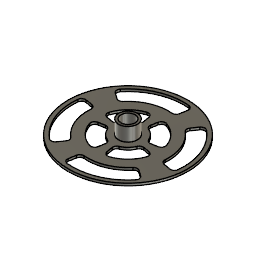
Holder 2 (Autodesk Fusion 360 design; units mm, degrees)
Autodesk Fusion 360 part; units mm, degrees
note: some values were not read from the file. Set by a fixed rule: which sketch regions a step uses.
sketch "Sketch1" plane through (0, 0, 0) normal (0, 0, 1) x (1, 0, 0)
  circle A0 centre (0, 0) radius 75
  circle A1 centre (0, 0) radius 46
  circle A2 centre (0, 0) radius 43
  circle A3 centre (0, 0) radius 11.9
  circle A4 centre (0, 0) radius 8.9
  line L0 (0, 90) -> (0, -90)
  line L1 (12.1554, 68.9365) -> (13.0236, 73.8606)
  line L2 (8.8561, 50.2252) -> (12.1554, 68.9365)
  line L3 (-12.1554, 68.9365) -> (-13.0236, 73.8606)
  line L4 (-8.8561, 50.2252) -> (-12.1554, 68.9365)
  arc A5 (-8.8561, 50.2252) -> (8.8561, 50.2252) centre (0, 0) ccw
  arc A6 (0, 51) -> (-8.8561, 50.2252) centre (0, 0) ccw
  arc A7 (8.8561, 50.2252) -> (0, 51) centre (0, 0) ccw
  arc A8 (-12.1554, 68.9365) -> (12.1554, 68.9365) centre (0, 0) ccw
  arc A9 (12.1554, 68.9365) -> (0, 70) centre (0, 0) ccw
  arc A10 (0, 70) -> (-12.1554, 68.9365) centre (0, 0) ccw
  arc A11 (-6.5986, 37.4227) -> (6.5986, 37.4227) centre (0, 0) ccw
  arc A12 (6.5986, 37.4227) -> (0, 38) centre (0, 0) ccw
  arc A13 (0, 38) -> (-6.5986, 37.4227) centre (0, 0) ccw
  line L5 (0, 0) -> (3.473, 19.6962)
  line L6 (6.5986, 37.4227) -> (8.8561, 50.2252)
  line L7 (3.473, 19.6962) -> (6.5986, 37.4227)
  line L8 (0, 0) -> (-3.473, 19.6962)
  line L9 (-6.5986, 37.4227) -> (-8.8561, 50.2252)
  line L10 (-3.473, 19.6962) -> (-6.5986, 37.4227)
  arc A14 (-3.473, 19.6962) -> (3.473, 19.6962) centre (0, 0) ccw
  arc A15 (0, 20) -> (-3.473, 19.6962) centre (0, 0) ccw
  arc A16 (3.473, 19.6962) -> (0, 20) centre (0, 0) ccw
  arc A17 (-40.1504, 57.3406) -> (-49.4975, 49.4975) centre (0, 0) ccw
  arc A18 (-49.4975, 49.4975) -> (-57.3406, 40.1504) centre (0, 0) ccw
  line L11 (-29.2524, 41.7768) -> (-40.1504, 57.3406)
  arc A19 (-29.2524, 41.7768) -> (-36.0624, 36.0624) centre (0, 0) ccw
  arc A20 (-36.0624, 36.0624) -> (-41.7768, 29.2524) centre (0, 0) ccw
  line L12 (-41.7768, 29.2524) -> (-57.3406, 40.1504)
  arc A21 (-21.7959, 31.1278) -> (-26.8701, 26.8701) centre (0, 0) ccw
  line L13 (-11.4715, 16.383) -> (-21.7959, 31.1278)
  arc A22 (-11.4715, 16.383) -> (-14.1421, 14.1421) centre (0, 0) ccw
  arc A23 (-14.1421, 14.1421) -> (-16.383, 11.4715) centre (0, 0) ccw
  line L14 (-16.383, 11.4715) -> (-31.1278, 21.7959)
  arc A24 (-26.8701, 26.8701) -> (-31.1278, 21.7959) centre (0, 0) ccw
  arc A25 (-68.9365, 12.1554) -> (-70, 0) centre (0, 0) ccw
  arc A26 (-70, 0) -> (-68.9365, -12.1554) centre (0, 0) ccw
  line L15 (-50.2252, 8.8561) -> (-68.9365, 12.1554)
  arc A27 (-50.2252, 8.8561) -> (-51, 0) centre (0, 0) ccw
  arc A28 (-51, 0) -> (-50.2252, -8.8561) centre (0, 0) ccw
  line L16 (-50.2252, -8.8561) -> (-68.9365, -12.1554)
  arc A29 (-37.4227, 6.5986) -> (-38, 0) centre (0, 0) ccw
  line L17 (-19.6962, 3.473) -> (-37.4227, 6.5986)
  arc A30 (-19.6962, 3.473) -> (-20, 0) centre (0, 0) ccw
  arc A31 (-20, 0) -> (-19.6962, -3.473) centre (0, 0) ccw
  line L18 (-19.6962, -3.473) -> (-37.4227, -6.5986)
  arc A32 (-38, 0) -> (-37.4227, -6.5986) centre (0, 0) ccw
  arc A33 (-57.3406, -40.1504) -> (-49.4975, -49.4975) centre (0, 0) ccw
  arc A34 (-49.4975, -49.4975) -> (-40.1504, -57.3406) centre (0, 0) ccw
  line L19 (-41.7768, -29.2524) -> (-57.3406, -40.1504)
  arc A35 (-41.7768, -29.2524) -> (-36.0624, -36.0624) centre (0, 0) ccw
  arc A36 (-36.0624, -36.0624) -> (-29.2524, -41.7768) centre (0, 0) ccw
  line L20 (-29.2524, -41.7768) -> (-40.1504, -57.3406)
  arc A37 (-31.1278, -21.7959) -> (-26.8701, -26.8701) centre (0, 0) ccw
  line L21 (-16.383, -11.4715) -> (-31.1278, -21.7959)
  arc A38 (-16.383, -11.4715) -> (-14.1421, -14.1421) centre (0, 0) ccw
  arc A39 (-14.1421, -14.1421) -> (-11.4715, -16.383) centre (0, 0) ccw
  line L22 (-11.4715, -16.383) -> (-21.7959, -31.1278)
  arc A40 (-26.8701, -26.8701) -> (-21.7959, -31.1278) centre (0, 0) ccw
  arc A41 (-12.1554, -68.9365) -> (0, -70) centre (0, 0) ccw
  arc A42 (0, -70) -> (12.1554, -68.9365) centre (0, 0) ccw
  line L23 (-8.8561, -50.2252) -> (-12.1554, -68.9365)
  arc A43 (-8.8561, -50.2252) -> (0, -51) centre (0, 0) ccw
  arc A44 (0, -51) -> (8.8561, -50.2252) centre (0, 0) ccw
  line L24 (8.8561, -50.2252) -> (12.1554, -68.9365)
  arc A45 (-6.5986, -37.4227) -> (0, -38) centre (0, 0) ccw
  line L25 (-3.473, -19.6962) -> (-6.5986, -37.4227)
  arc A46 (-3.473, -19.6962) -> (0, -20) centre (0, 0) ccw
  arc A47 (0, -20) -> (3.473, -19.6962) centre (0, 0) ccw
  line L26 (3.473, -19.6962) -> (6.5986, -37.4227)
  arc A48 (0, -38) -> (6.5986, -37.4227) centre (0, 0) ccw
  arc A49 (40.1504, -57.3406) -> (49.4975, -49.4975) centre (0, 0) ccw
  arc A50 (49.4975, -49.4975) -> (57.3406, -40.1504) centre (0, 0) ccw
  line L27 (29.2524, -41.7768) -> (40.1504, -57.3406)
  arc A51 (29.2524, -41.7768) -> (36.0624, -36.0624) centre (0, 0) ccw
  arc A52 (36.0624, -36.0624) -> (41.7768, -29.2524) centre (0, 0) ccw
  line L28 (41.7768, -29.2524) -> (57.3406, -40.1504)
  arc A53 (21.7959, -31.1278) -> (26.8701, -26.8701) centre (0, 0) ccw
  line L29 (11.4715, -16.383) -> (21.7959, -31.1278)
  arc A54 (11.4715, -16.383) -> (14.1421, -14.1421) centre (0, 0) ccw
  arc A55 (14.1421, -14.1421) -> (16.383, -11.4715) centre (0, 0) ccw
  line L30 (16.383, -11.4715) -> (31.1278, -21.7959)
  arc A56 (26.8701, -26.8701) -> (31.1278, -21.7959) centre (0, 0) ccw
  arc A57 (68.9365, -12.1554) -> (70, 0) centre (0, 0) ccw
  arc A58 (70, 0) -> (68.9365, 12.1554) centre (0, 0) ccw
  line L31 (50.2252, -8.8561) -> (68.9365, -12.1554)
  arc A59 (50.2252, -8.8561) -> (51, 0) centre (0, 0) ccw
  arc A60 (51, 0) -> (50.2252, 8.8561) centre (0, 0) ccw
  line L32 (50.2252, 8.8561) -> (68.9365, 12.1554)
  arc A61 (37.4227, -6.5986) -> (38, 0) centre (0, 0) ccw
  line L33 (19.6962, -3.473) -> (37.4227, -6.5986)
  arc A62 (19.6962, -3.473) -> (20, 0) centre (0, 0) ccw
  arc A63 (20, 0) -> (19.6962, 3.473) centre (0, 0) ccw
  line L34 (19.6962, 3.473) -> (37.4227, 6.5986)
  arc A64 (38, 0) -> (37.4227, 6.5986) centre (0, 0) ccw
  arc A65 (57.3406, 40.1504) -> (49.4975, 49.4975) centre (0, 0) ccw
  arc A66 (49.4975, 49.4975) -> (40.1504, 57.3406) centre (0, 0) ccw
  line L35 (41.7768, 29.2524) -> (57.3406, 40.1504)
  arc A67 (41.7768, 29.2524) -> (36.0624, 36.0624) centre (0, 0) ccw
  arc A68 (36.0624, 36.0624) -> (29.2524, 41.7768) centre (0, 0) ccw
  line L36 (29.2524, 41.7768) -> (40.1504, 57.3406)
  arc A69 (31.1278, 21.7959) -> (26.8701, 26.8701) centre (0, 0) ccw
  line L37 (16.383, 11.4715) -> (31.1278, 21.7959)
  arc A70 (16.383, 11.4715) -> (14.1421, 14.1421) centre (0, 0) ccw
  arc A71 (14.1421, 14.1421) -> (11.4715, 16.383) centre (0, 0) ccw
  line L38 (11.4715, 16.383) -> (21.7959, 31.1278)
  arc A72 (26.8701, 26.8701) -> (21.7959, 31.1278) centre (0, 0) ccw
  dimension "d1" = 150
  dimension "d2" = -29
  dimension "d3" = -3
  dimension "d12" = 23.8
  dimension "d13" = -3
  dimension "d20" = 10
  dimension "d21" = 20
  dimension "d23" = 360
  constraint coincident A0.centre A1.centre
  constraint concentric A0 A3
  constraint vertical L0
  constraint coincident A0.centre L0
  constraint coincident A0 L1.end
  constraint coincident A0 L3.end
  constraint concentric A1 A5
  constraint coincident L0 A6.start
  constraint concentric A5 A6
  constraint concentric A5 A7
  constraint concentric A0 A8
  constraint coincident L0 A9.end
  constraint concentric A8 A9
  constraint concentric A8 A10
  constraint concentric A2 A11
  constraint coincident A11.end L5
  constraint coincident L0 A12.end
  constraint concentric A11 A12
  constraint coincident A11.start L8
  constraint concentric A11 A13
  constraint concentric A3 A14
  constraint coincident L0 A15.start
  constraint concentric A14 A15
  constraint concentric A14 A16
  measures "d1" diameter of A0
  measures "d12" diameter of A3
  measures "d20" angle of L0 L8
  measures "d21" angle of L5 L8
extrude "Extrude1" add sketch "Sketch1" along normal blind 3
extrude "Extrude3" add sketch "Sketch1" along normal blind 20 contours A3 A4 L0 L5 | A3 A4 L0 L5 | A3 A4 L0 L8 | A3 A4 L0 L8
extrude "Extrude4" cut sketch "Sketch1" along normal up to surface (3 mm away) contours L0 L2 A7 A9 | L0 A5 A8 A41 L23 A43 | L0 A5 A8 A42 A44 L24 | L0 L4 A6 A10 | A5 A8 A65 A66 L35 A67 A68 L36 | L4 A5 A8 L11 | A5 A8 L24 L27 | A5 A8 A17 A18 L11 A19 A20 L12 | A5 A8 A33 A34 L19 A35 A36 L20 | A5 A8 A49 A50 L27 A51 A52 L28 | A5 A8 L32 L35 | A5 A8 A57 A58 L31 A59 A60 L32 | A5 A8 L16 L19 | A5 A8 A25 A26 L15 A27 A28 L16
fillet "Fillet5" radius 5 16 edges at (-68.9365, 12.1554, 1.5) (-50.2252, 8.8561, 1.5) (-40.1504, -57.3406, 1.5) (-29.2524, -41.7768, 1.5) (-12.1554, -68.9365, 1.5) (-8.8561, -50.2252, 1.5) (57.3406, -40.1504, 1.5) (41.7768, -29.2524, 1.5) (68.9365, -12.1554, 1.5) (50.2252, -8.8561, 1.5) (40.1504, 57.3406, 1.5) (29.2524, 41.7768, 1.5) (8.8561, 50.2252, 1.5) (12.1554, 68.9365, 1.5) (-57.3406, 40.1504, 1.5) (-41.7768, 29.2524, 1.5)
extrude "Extrude5" cut sketch "Sketch1" along normal up to surface (3 mm away) contours A11 L7 A14 L38 | A11 A14 A69 L37 A70 A71 L38 A72 | A11 L10 A14 L13 | A11 A14 L22 L25 | A11 A14 L26 L29 | A11 A14 A21 L13 A22 A23 L14 A24 | A11 A14 A37 L21 A38 A39 L22 A40 | A11 A14 A53 L29 A54 A55 L30 A56 | A11 A14 L34 L37 | A11 A14 L14 L17 | A11 A14 L18 L21 | A11 A14 L30 L33
fillet "Fillet6" radius 5 16 edges at (-6.5986, 37.4227, 1.5) (-3.473, 19.6962, 1.5) (-37.4227, 6.5986, 1.5) (-19.6962, 3.473, 1.5) (-37.4227, -6.5986, 1.5) (-19.6962, -3.473, 1.5) (-6.5986, -37.4227, 1.5) (-3.473, -19.6962, 1.5) (6.5986, -37.4227, 1.5) (3.473, -19.6962, 1.5) (19.6962, -3.473, 1.5) (37.4227, -6.5986, 1.5) (37.4227, 6.5986, 1.5) (19.6962, 3.473, 1.5) (6.5986, 37.4227, 1.5) (3.473, 19.6962, 1.5)
